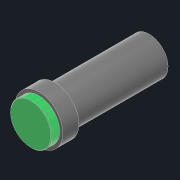
# Autodesk Inventor part: AP6MS54G
Saved by Autodesk Inventor 2022 (Build 260153000, 153)
## iProperties
Created: 2021-07-24
Part Number: AP6MS54G
Material: ABS プラスチック
Document SubType Name: Modeling
Designer: yuta0
Density: 1.06 g/cm^3
Appearance: 滑らか - 黒
Description: Amazon
購入先: Amazon
在庫数: 0.0
Author: yuta0
Autodesk Inventor part; units mm, degrees
ref_plane "YZ Plane" through (0, 0, 0) normal (1, 0, 0) x (0, 1, 0)
ref_plane "XZ Plane" through (0, 0, 0) normal (0, 1, 0) x (-1, 0, 0)
ref_plane "XY Plane" through (0, 0, 0) normal (0, 0, 1) x (1, 0, 0)
sketch "スケッチ1" plane through (0, 0, 0) normal (1, 0, 0) x (0, 1, 0)
  line L0 (8.9, -3) -> (8.9, -9)
  line L1 (8.9, -9) -> (7, -9)
  line L2 (7, -9) -> (7, -44)
  line L3 (7, -44) -> (0, -44)
  line L4 (0, -44) -> (0, 0)
  line L5 (8.9, -3) -> (7.7, -3)
  line L6 (7.7, -3) -> (7.7, 0)
  line L7 (7.7, 0) -> (0, 0)
  dimension "d0" = 8.9
  dimension "d1" = 3
  dimension "d2" = 9
  dimension "d4" = 7.7
  dimension "d5" = 7
  dimension "d10" = 35
  constraints: 16 end point, 7 perpendicular, 1 horizontal
  measures "d0" distance between parallel lines of L4 L0
  measures "d1" distance of L5.end L6.end
  measures "d2" distance between parallel lines of L7 L1
  measures "d4" distance of L6.end L4.end
  measures "d5" distance between parallel lines of L4 L2
  measures "d10" distance of L1.end L2.end
revolve "回転1" add sketch "スケッチ1" angle 360 about axis through (0, 0, -44) along (0, 0, 1)
chamfer "面取り1" distance 0.2 angle 45 1 edges at (0, -7.7, 0)
